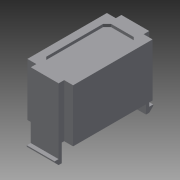
# Autodesk Inventor part: motor_shaft
Saved by Autodesk Inventor 2014 (Build 180170000, 170)
## iProperties
Created: 2013-06-25
Part Number: motor_shaft
Material: Generisch
Document SubType Name: Modeling
Designer: Felix
Density: 1 g/cm^3
Appearance: Vorgabe
Author: Felix
Autodesk Inventor part; units mm, degrees
ref_plane "YZ Plane" through (0, 0, 0) normal (1, 0, 0) x (0, 1, 0)
ref_plane "XZ Plane" through (0, 0, 0) normal (0, 1, 0) x (-1, 0, 0)
sketch "Skizze1" plane through (0, 0, 0) normal (0, 0, 1) x (1, 0, 0)
  line L0 (0, 0) -> (11.5, 0)
  line L1 (11.5, 0) -> (11.5, 20)
  line L2 (11.5, 20) -> (0, 20)
  line L3 (0, 20) -> (0, 0)
  line L4 (2.25, 20) -> (9.25, 20)
  line L5 (9.25, 20) -> (9.25, 21.4)
  line L6 (9.25, 21.4) -> (2.25, 21.4)
  line L7 (2.25, 21.4) -> (2.25, 20)
  line L8 (2.2583, 0) -> (10.4927, 0)
  line L9 (9.25, 0) -> (2.25, 0)
  line L10 (2.25, 0) -> (2.25, -1.4)
  line L11 (2.25, -1.4) -> (9.25, -1.4)
  line L12 (9.25, -1.4) -> (9.25, 0)
  dimension "d0" = 11.5
  dimension "d1" = 20
  dimension "d4" = 7
  dimension "d5" = 1.4
  dimension "d6" = 2.25
  dimension "d7" = 2.25
  constraints: 26 end point, 6 parallel, 4 horizontal, 3 perpendicular, 3 point on line, 2 equal length
  measures "d0" distance of L2.end L1.end
  measures "d1" distance of L1.end L0.end
  measures "d4" distance of L5.end L6.end
  measures "d5" distance of L4.end L5.end
  measures "d6" distance between parallel lines of L3 L7
  measures "d7" distance between parallel lines of L3 L10
extrude "Extrusion1" add sketch "Skizze1" along normal blind 13.3
ref_plane "Arbeitsebene2" through (2.25, 10, 0) normal (0, 1, 0) x (1, 0, 0)
sketch "Skizze2" plane through (0, 0, 13.3) normal (0, 0, 1) x (1, 0, 0)
  line L0 (9.25, 21.4) -> (2.25, 21.4) projected
  line L1 (0, 20) -> (0, 0) projected
  line L2 (2.25, -1.4) -> (9.25, -1.4) projected
  line L3 (11.5, 0) -> (11.5, 20) projected
  line L4 (2.9, 18.15) -> (8.6, 18.15)
  line L5 (9.6, 17.15) -> (9.6, 2.85)
  line L6 (8.6, 1.85) -> (2.9, 1.85)
  line L7 (1.9, 2.85) -> (1.9, 17.15)
  line L8 (2.9, 18.15) -> (1.9, 17.15)
  line L9 (8.6, 18.15) -> (9.6, 17.15)
  line L10 (9.6, 2.85) -> (8.6, 1.85)
  line L11 (2.9, 1.85) -> (1.9, 2.85)
  point P0 (1.9, 18.15)
  point P1 (9.6, 1.85)
  point P2 (9.6, 18.15)
  point P3 (1.9, 1.85)
  dimension "d8" = 1.9
  dimension "d9" = 1.9
  dimension "d10" = 3.25
  dimension "d11" = 3.25
  dimension "d12" = 1
  dimension "d13" = 1
  dimension "d14" = 1
  dimension "d15" = 1
  dimension "d16" = 1
  dimension "d17" = 1
  dimension "d18" = 1
  dimension "d19" = 1
  constraints: 16 end point, 8 point on line, 2 parallel, 1 horizontal, 1 perpendicular
  measures "d8" distance between parallel lines of L7 L1
  measures "d9" distance between parallel lines of L5 L3
  measures "d10" distance between parallel lines of L0 L4
  measures "d11" distance between parallel lines of L6 L2
  measures "d12" distance of L4.start point (1.9, 18.15)
  measures "d13" distance of L7.end point (1.9, 18.15)
  measures "d14" distance of L4.end point (9.6, 18.15)
  measures "d15" distance of L5.start point (9.6, 18.15)
  measures "d16" distance of L5.end point (9.6, 1.85)
  measures "d17" distance of L6.start point (9.6, 1.85)
  measures "d18" distance of L6.end point (1.9, 1.85)
  measures "d19" distance of L7.start point (1.9, 1.85)
extrude "Extrusion2" cut sketch "Skizze2" against normal blind 0.7
sketch "Skizze4" plane through (0, 0, 0) normal (0, 0, -1) x (-1, 0, 0)
  line L0 (-2.25, 21.4) -> (-2.25, 20) projected
  line L1 (-9.25, 21.4) -> (-2.25, 21.4) projected
  line L2 (-9.25, 20) -> (-9.25, 21.4) projected
  line L3 (-9.25, -1.4) -> (-9.25, 0) projected
  line L4 (-2.25, -1.4) -> (-9.25, -1.4) projected
  line L5 (-2.25, 0) -> (-2.25, -1.4) projected
  line L6 (-9.25, 20.6) -> (-2.25, 20.6)
  dimension "d32" = 0.8
  constraints: 2 end point, 2 point on line, 1 perpendicular
  measures "d32" distance between parallel lines of L1 L6
extrude "Extrusion3" add sketch "Skizze4" along normal blind 4.5
sketch "Skizze5" plane through (2.25, 21.4, 13.3) normal (0, 1, 0) x (1, 0, 0)
  line L0 (7, 17.8) -> (7, 0) projected
  line L1 (0, 17.8) -> (7, 17.8) projected
  line L2 (0, 17.8) -> (7, 17.8)
  line L3 (7, 17.8) -> (7, 16.5)
  line L4 (7, 16.5) -> (0, 16.5)
  line L5 (0, 16.5) -> (0, 17.8)
  point P0 (-2.25, 13.3)
  dimension "d36" = 1.3
  constraints: 8 end point, 2 parallel, 1 horizontal, 1 perpendicular, 1 point on line
  measures "d36" distance between parallel lines of L2 L4
extrude "Extrusion4" add sketch "Skizze5" along normal blind 1
chamfer "Fase1" distance 1 angle 45 1 edges at (5.75, 22.4, -4.5)
mirror "Spiegeln1" about plane through (2.25, 10, 0) normal (0, 1, 0) of "Extrusion4", "Fase1", "Extrusion3"
equation "\"d13\" = d12"
equation "\"d14\" = d12"
equation "\"d15\" = d14"
equation "\"d16\" = d12"
equation "\"d17\" = d16"
equation "\"d18\" = d12"
equation "\"d19\" = d18"
